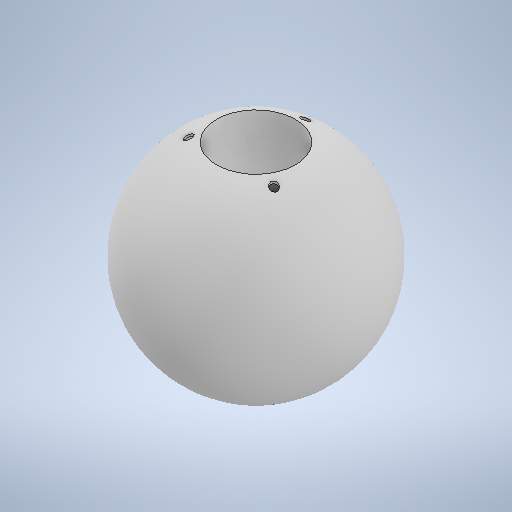
# Autodesk Inventor part: Buoy 7 TallShpere
Saved by Autodesk Inventor 2025 (Build 290162000, 162)
## iProperties
Created: 2024-06-27
Part Number: Buoy 7 TallShpere
Material: Generic
Document SubType Name: Modeling
Designer: track
Density: 1 g/cm^3
Appearance: Default
Author: track
Autodesk Inventor part; units mm, degrees
ref_plane "YZ Plane" through (0, 0, 0) normal (1, 0, 0) x (0, 1, 0)
ref_plane "XZ Plane" through (0, 0, 0) normal (0, 1, 0) x (-1, 0, 0)
ref_plane "XY Plane" through (0, 0, 0) normal (0, 0, 1) x (1, 0, 0)
sketch "Sketch1" plane through (0, 0, 0) normal (0, 0, 1) x (1, 0, 0)
  line L0 (0, 0) -> (0, 152.4) construction
  line L1 (0, 152.4) -> (30.48, 152.4) construction
  line L2 (30.48, 152.4) -> (30.48, 0)
  arc A0 (30.48, 0) -> (30.48, 152.4) centre (-1.27, 76.2) ccw
  line L3 (31.98, 2.2842) -> (31.98, 150.1158)
  arc A1 (31.98, 2.2842) -> (31.98, 150.1158) centre (-1.27, 76.2) ccw
  dimension "d0" = 152.4
  dimension "d1" = 152.4
  dimension "d2" = 30.48
  dimension "d3" = 82.55
  dimension "d4" = 1.5
  constraints: 8 end point, 4 point on circle, 2 centre point, 2 perpendicular, 1 vertical, 1 other
  measures "d0" distance of L0.start L0.end
  measures "d1" distance of L1.end L2.end
  measures "d2" distance between parallel lines of L0 L2
  measures "d3" radius of A0
  measures "d4" radial gap between concentric circles of A0 A1
revolve "Revolution1" add sketch "Sketch1" angle 360 about axis through (0, 0, 0) along (0, 1, 0)
sketch "Sketch2" plane through (0, 0, 0) normal (0, 1, 0) x (-1, 0, 0)
  line L0 (0, 0) -> (0, -38.1) construction
  circle A0 centre (0, -38.1) radius 3
  dimension "d6" = 38.1
  dimension "d7" = 6
  constraints: 2 end point, 1 centre point, 1 coincident, 1 vertical
  measures "d6" distance of L0.start L0.end
  measures "d7" diameter of A0
extrude "Extrusion1" cut sketch "Sketch2" along normal blind 152.4
pattern_circular "Circular Pattern1" count 3 over 360 about axis through (0, 76.2, 0) along (0, 1, 0) of "Extrusion1"
body "Solid1"
